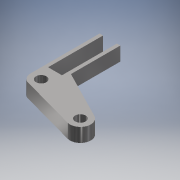
# Autodesk Inventor part: steeringarm
Saved by Autodesk Inventor 2018 (Build 220112000, 112)
## iProperties
Created: 2018-08-06
Part Number: steeringarm
Material: Steel, Mild
Document SubType Name: Modeling
Designer: Cole Tucker
Density: 7.85 g/cm^3
Appearance: Semi-Polished
Mass: 172.965 g
Surface Area: 89.1037 cm^2
Volume: 22.0337 cm^3
Author: Cole Tucker
Autodesk Inventor part; units mm, degrees
ref_plane "YZ Plane" through (0, 0, 0) normal (1, 0, 0) x (0, 1, 0)
ref_plane "XZ Plane" through (0, 0, 0) normal (0, 1, 0) x (-1, 0, 0)
ref_plane "XY Plane" through (0, 0, 0) normal (0, 0, 1) x (1, 0, 0)
sketch "Sketch1" plane through (0, 0, 0) normal (0, 1, 0) x (-1, 0, 0)
  circle A0 centre (0, 0) radius 6.35
  line L0 (0, 0) -> (12.7, 0) construction
  line L1 (12.7, 0) -> (12.7, -12.7) construction
  line L2 (12.7, -12.7) -> (0, -12.7) construction
  line L3 (0, -12.7) -> (0, 0) construction
  line L4 (0, 0) -> (0, 130.5863) construction
  line L5 (0, 0) -> (-25.4, 0) construction
  line L6 (0, 0) -> (26.296, 98.1381) construction
  circle A1 centre (26.296, 98.1381) radius 4.7625
  line L7 (-76.2, -6.35) -> (-25.4, -6.35)
  line L8 (-25.4, -6.35) -> (-25.4, 0)
  line L9 (-76.2, 6.35) -> (-25.4, 6.35)
  line L10 (-25.4, 6.35) -> (-25.4, 0)
  circle A2 centre (26.296, 98.1381) radius 9.525
  line L11 (35.4965, 95.6728) -> (12.7, -12.7)
  line L12 (0, 0) -> (-12.7, 0) construction
  line L13 (-12.7, 0) -> (-12.7, 12.7) construction
  line L14 (-12.7, 12.7) -> (0, 12.7) construction
  line L15 (0, 12.7) -> (0, 0) construction
  line L16 (-12.7, 12.7) -> (17.0956, 100.6033)
  line L17 (-76.2, 6.35) -> (-76.2, 12.7)
  line L18 (-76.2, 12.7) -> (-12.7, 12.7)
  line L19 (-76.2, -6.35) -> (-76.2, -12.7)
  line L20 (-76.2, -12.7) -> (12.7, -12.7)
  dimension "d18" = 12.7
  dimension "d19" = 12.7
  dimension "d20" = 12.7
  dimension "d21" = 25.4
  dimension "d22" = 101.6
  dimension "d23" = 15
  dimension "d24" = 9.525
  dimension "d25" = 50.8
  dimension "d27" = 50.8
  dimension "d29" = 19.05
  dimension "d30" = 12.7
  dimension "d31" = 12.7
  dimension "d32" = 6.35
  dimension "d33" = 6.35
  dimension "d34" = 12.7
  dimension "d35" = 88.9
  constraints: 42 end point, 4 parallel, 3 centre point, 3 horizontal, 2 coincident, 2 perpendicular, 2 point on circle, 2 vertical, 1 point on line
  measures "d18" diameter of A0
  measures "d19" distance of L1.end L2.end
  measures "d20" distance of L0.end L1.end
  measures "d21" distance of L0.start L5.end
  measures "d22" distance of L0.start L6.end
  measures "d23" angle of L4 L6
  measures "d24" diameter of A1
  measures "d25" distance of L7.end L7.start
  measures "d27" distance of L9.start L9.end
  measures "d29" diameter of A2
  measures "d30" distance of L13.end L14.end
  measures "d31" distance of L12.end L13.end
  measures "d32" distance of L9.start L17.end
  measures "d33" distance of L7.start L19.end
  measures "d34" distance between parallel lines of L9 L7
  measures "d35" distance of L19.end L1.end
extrude "Extrusion3" add sketch "Sketch1" along normal blind 12.7
fillet "Fillet2" radius 12.7 2 edges at (12.7, 6.35, 12.7) (-12.7, 6.35, -12.7)
body "Solid3"
